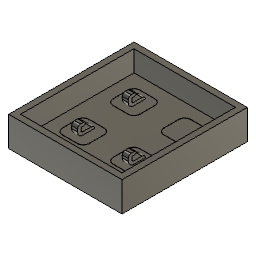
Modular key holder (Autodesk Fusion 360 design; units mm, degrees)
Autodesk Fusion 360 part; units mm, degrees
sketch "Sketch1" plane through (0, 0, 0) normal (0, 0, 1) x (1, 0, 0)
  line L0 (0, 0) -> (190, 0)
  line L1 (190, 0) -> (190, 210)
  line L2 (190, 210) -> (0, 210)
  line L3 (0, 210) -> (0, 0)
  line L4 (10, 10) -> (180, 10)
  line L5 (180, 10) -> (180, 200)
  line L6 (180, 200) -> (10, 200)
  line L7 (10, 200) -> (10, 10)
  dimension "d1" = 190
  dimension "d2" = 210
  dimension "d3" = -10
  constraint horizontal L0
  constraint vertical L1
  constraint horizontal L2
  constraint vertical L3
  constraint coincident L0.start L3.end
  measures "d1" distance of L0.start L0.end
  measures "d2" distance of L0.start L2.end
extrude "Extrude1" add sketch "Sketch1" along normal blind 50 makes body 1
extrude "Extrude2" add sketch "Sketch1" along normal blind 15 contours L4 L5 L6 L7 bodies 1
sketch "Sketch2" plane through (0, 0, 0) normal (0, 0, -1) x (1, 0, 0)
  line L0 (0, 0) -> (0, -210)
  line L1 (0, -210) -> (190, -210)
  line L2 (190, -210) -> (190, 0)
  line L3 (190, 0) -> (0, 0)
  line L4 (170, -160) -> (20, -160)
  line L5 (20, -160) -> (20, -145)
  line L6 (20, -145) -> (170, -145)
  line L7 (170, -145) -> (170, -160)
  dimension "d10" = 150
  dimension "d11" = 15
  constraint horizontal L4
  constraint vertical L5
  constraint horizontal L6
  constraint vertical L7
  measures "d10" distance of L4.start L4.end
  measures "d11" distance of L4.start L6.end
extrude "Extrude3" cut sketch "Sketch2" against normal blind 7 contours L4 L5 L6 L7 bodies 1
sketch "Sketch3" plane through (0, 0, 7) normal (0, 0, -1) x (1, 0, 0)
  line L0 (170, -145) -> (20, -145)
  line L1 (20, -145) -> (20, -160)
  line L2 (20, -160) -> (170, -160)
  line L3 (170, -160) -> (170, -145)
  spline S0 degree 2 poles (16.5, -160) (20.152, -154.0538) (23.5, -160) knots 0 0 0 1.133962 1.133962 1.133962 weights 1 3 1
  spline S1 degree 2 poles (23.0217, -160) (26.6738, -154.0538) (30.0217, -160) knots 0 0 0 1.133962 1.133962 1.133962 weights 1 3 1
  spline S2 degree 2 poles (29.5435, -160) (33.1955, -154.0538) (36.5435, -160) knots 0 0 0 1.133962 1.133962 1.133962 weights 1 3 1
  spline S3 degree 2 poles (36.0652, -160) (39.7173, -154.0538) (43.0652, -160) knots 0 0 0 1.133962 1.133962 1.133962 weights 1 3 1
  spline S4 degree 2 poles (42.587, -160) (46.239, -154.0538) (49.587, -160) knots 0 0 0 1.133962 1.133962 1.133962 weights 1 3 1
  spline S5 degree 2 poles (49.1087, -160) (52.7607, -154.0538) (56.1087, -160) knots 0 0 0 1.133962 1.133962 1.133962 weights 1 3 1
  spline S6 degree 2 poles (55.6304, -160) (59.2825, -154.0538) (62.6304, -160) knots 0 0 0 1.133962 1.133962 1.133962 weights 1 3 1
  spline S7 degree 2 poles (62.1522, -160) (65.8042, -154.0538) (69.1522, -160) knots 0 0 0 1.133962 1.133962 1.133962 weights 1 3 1
  spline S8 degree 2 poles (68.6739, -160) (72.326, -154.0538) (75.6739, -160) knots 0 0 0 1.133962 1.133962 1.133962 weights 1 3 1
  spline S9 degree 2 poles (75.1957, -160) (78.8477, -154.0538) (82.1957, -160) knots 0 0 0 1.133962 1.133962 1.133962 weights 1 3 1
  spline S10 degree 2 poles (81.7174, -160) (85.3694, -154.0538) (88.7174, -160) knots 0 0 0 1.133962 1.133962 1.133962 weights 1 3 1
  spline S11 degree 2 poles (88.2391, -160) (91.8912, -154.0538) (95.2391, -160) knots 0 0 0 1.133962 1.133962 1.133962 weights 1 3 1
  spline S12 degree 2 poles (94.7609, -160) (98.4129, -154.0538) (101.7609, -160) knots 0 0 0 1.133962 1.133962 1.133962 weights 1 3 1
  spline S13 degree 2 poles (101.2826, -160) (104.9347, -154.0538) (108.2826, -160) knots 0 0 0 1.133962 1.133962 1.133962 weights 1 3 1
  spline S14 degree 2 poles (107.8043, -160) (111.4564, -154.0538) (114.8043, -160) knots 0 0 0 1.133962 1.133962 1.133962 weights 1 3 1
  spline S15 degree 2 poles (114.3261, -160) (117.9781, -154.0538) (121.3261, -160) knots 0 0 0 1.133962 1.133962 1.133962 weights 1 3 1
  spline S16 degree 2 poles (120.8478, -160) (124.4999, -154.0538) (127.8478, -160) knots 0 0 0 1.133962 1.133962 1.133962 weights 1 3 1
  spline S17 degree 2 poles (127.3696, -160) (131.0216, -154.0538) (134.3696, -160) knots 0 0 0 1.133962 1.133962 1.133962 weights 1 3 1
  spline S18 degree 2 poles (133.8913, -160) (137.5433, -154.0538) (140.8913, -160) knots 0 0 0 1.133962 1.133962 1.133962 weights 1 3 1
  spline S19 degree 2 poles (140.413, -160) (144.0651, -154.0538) (147.413, -160) knots 0 0 0 1.133962 1.133962 1.133962 weights 1 3 1
  spline S20 degree 2 poles (146.9348, -160) (150.5868, -154.0538) (153.9348, -160) knots 0 0 0 1.133962 1.133962 1.133962 weights 1 3 1
  spline S21 degree 2 poles (153.4565, -160) (157.1086, -154.0538) (160.4565, -160) knots 0 0 0 1.133962 1.133962 1.133962 weights 1 3 1
  spline S22 degree 2 poles (159.9783, -160) (163.6303, -154.0538) (166.9783, -160) knots 0 0 0 1.133962 1.133962 1.133962 weights 1 3 1
  spline S23 degree 2 poles (166.5, -160) (170.152, -154.0538) (173.5, -160) knots 0 0 0 1.133962 1.133962 1.133962 weights 1 3 1
  dimension "d18" = 0
  dimension "d19" = -150
extrude "Extrude4" add sketch "Sketch3" along normal blind 2 from surface at 5 contours L2 L3 S22 S23 | L1 L2 S0 S1 | L2 S21 S22 S23 | L2 S22 S23 | L2 S0 S1 S2 | L2 S0 S1 | L2 S20 S21 S22 | L2 S21 S22 | L2 S1 S2 S3 | L2 S1 S2 | L2 S19 S20 S21 | L2 S20 S21 | L2 S2 S3 S4 | L2 S2 S3 | L2 S18 S19 S20 | L2 S19 S20 | L2 S3 S4 S5 | L2 S3 S4 | L2 S17 S18 S19 | L2 S18 S19 | L2 S4 S5 S6 | L2 S4 S5 | L2 S16 S17 S18 | L2 S17 S18 | L2 S5 S6 S7 | L2 S5 S6 | L2 S15 S16 S17 | L2 S16 S17 | L2 S6 S7 S8 | L2 S6 S7 | L2 S14 S15 S16 | L2 S15 S16 | L2 S7 S8 S9 | L2 S7 S8 | L2 S13 S14 S15 | L2 S14 S15 | L2 S8 S9 S10 | L2 S8 S9 | L2 S12 S13 S14 | L2 S13 S14 | L2 S9 S10 S11 | L2 S9 S10 | L2 S11 S12 S13 | L2 S12 S13 | L2 S10 S11 S12 | L2 S10 S11 | L2 S11 S12 bodies 1
sketch "Sketch4" plane through (0, 0, 15) normal (0, 0, 1) x (-1, 0, 0)
  line L0 (-10, -200) -> (-10, -10)
  line L1 (-10, -10) -> (-180, -10)
  line L2 (-180, -10) -> (-180, -200)
  line L3 (-180, -200) -> (-10, -200)
  line L4 (-40, -180) -> (-65, -180)
  line L5 (-75, -170) -> (-75, -145)
  line L6 (-65, -135) -> (-40, -135)
  line L7 (-30, -145) -> (-30, -170)
  line L8 (-150, -180) -> (-125, -180)
  line L9 (-115, -170) -> (-115, -145)
  line L10 (-125, -135) -> (-150, -135)
  line L11 (-160, -145) -> (-160, -170)
  line L12 (-40, -95) -> (-65, -95)
  line L13 (-75, -85) -> (-75, -60)
  line L14 (-65, -50) -> (-40, -50)
  line L15 (-30, -60) -> (-30, -85)
  line L16 (-150, -95) -> (-125, -95)
  line L17 (-115, -85) -> (-115, -60)
  line L18 (-160, -60) -> (-160, -85)
  line L19 (-125, -50) -> (-150, -50)
  arc A0 (-40, -180) -> (-30, -170) centre (-40, -170) ccw
  arc A1 (-75, -170) -> (-65, -180) centre (-65, -170) ccw
  arc A2 (-65, -135) -> (-75, -145) centre (-65, -145) ccw
  arc A3 (-30, -145) -> (-40, -135) centre (-40, -145) ccw
  arc A4 (-125, -180) -> (-115, -170) centre (-125, -170) ccw
  arc A5 (-160, -170) -> (-150, -180) centre (-150, -170) ccw
  arc A6 (-150, -135) -> (-160, -145) centre (-150, -145) ccw
  arc A7 (-115, -145) -> (-125, -135) centre (-125, -145) ccw
  arc A8 (-125, -95) -> (-115, -85) centre (-125, -85) ccw
  arc A9 (-160, -85) -> (-150, -95) centre (-150, -85) ccw
  arc A10 (-150, -50) -> (-160, -60) centre (-150, -60) ccw
  arc A11 (-115, -60) -> (-125, -50) centre (-125, -60) ccw
  arc A12 (-65, -50) -> (-75, -60) centre (-65, -60) ccw
  arc A13 (-30, -60) -> (-40, -50) centre (-40, -60) ccw
  arc A14 (-75, -85) -> (-65, -95) centre (-65, -85) ccw
  arc A15 (-40, -95) -> (-30, -85) centre (-40, -85) ccw
  point P0 (-30, -180)
  point P1 (-75, -180)
  point P2 (-30, -135)
  point P3 (-160, -180)
  point P4 (-115, -180)
  point P5 (-160, -135)
  point P6 (-160, -95)
  point P7 (-30, -50)
  point P8 (-115, -95)
  point P9 (-160, -50)
  point P10 (-30, -95)
  point P11 (-75, -95)
  dimension "d27" = 45
  dimension "d28" = 45
  dimension "d29" = 45
  dimension "d30" = 45
  dimension "d31" = 45
  dimension "d32" = 45
  dimension "d33" = 45
  dimension "d34" = 45
  dimension "d35" = 10
  constraint horizontal L4
  constraint vertical L5
  constraint horizontal L6
  constraint vertical L7
  constraint horizontal L8
  constraint vertical L9
  constraint horizontal L10
  constraint vertical L11
  constraint horizontal L12
  constraint vertical L13
  constraint horizontal L14
  constraint vertical L15
  constraint horizontal L16
  constraint vertical L17
  constraint horizontal L19
  constraint vertical L18
  constraint coincident P0 L4
  constraint coincident P0 L7
  constraint tangent L4 A0
  constraint tangent L7 A0
  constraint coincident P1 L4
  constraint coincident P1 L5
  constraint tangent L4 A1
  constraint tangent L5 A1
  constraint equal A0 A1
  constraint tangent L5 A2
  constraint tangent L6 A2
  constraint equal A0 A2
  constraint coincident P2 L6
  constraint coincident P2 L7
  constraint tangent L6 A3
  constraint tangent L7 A3
  constraint equal A0 A3
  constraint coincident P4 L8
  constraint coincident P4 L9
  constraint tangent L8 A4
  constraint tangent L9 A4
  constraint equal A0 A4
  constraint coincident P3 L8
  constraint coincident P3 L11
  constraint tangent L8 A5
  constraint tangent L11 A5
  constraint equal A0 A5
  constraint coincident P5 L10
  constraint coincident P5 L11
  constraint tangent L10 A6
  constraint tangent L11 A6
  constraint equal A0 A6
  constraint tangent L9 A7
  constraint tangent L10 A7
  constraint equal A0 A7
  constraint coincident P8 L16
  constraint coincident P8 L17
  constraint tangent L16 A8
  constraint tangent L17 A8
  constraint equal A0 A8
  constraint coincident P6 L16
  constraint coincident P6 L18
  constraint tangent L16 A9
  constraint tangent L18 A9
  constraint equal A0 A9
  constraint coincident P9 L18
  constraint coincident P9 L19
  constraint tangent L18 A10
  constraint tangent L19 A10
  constraint equal A0 A10
  constraint tangent L17 A11
  constraint tangent L19 A11
  constraint equal A0 A11
  constraint tangent L13 A12
  constraint tangent L14 A12
  constraint equal A0 A12
  constraint coincident P7 L14
  constraint coincident P7 L15
  constraint tangent L14 A13
  constraint tangent L15 A13
  constraint equal A0 A13
  constraint coincident P11 L12
  constraint coincident P11 L13
  constraint tangent L12 A14
  constraint tangent L13 A14
  constraint equal A0 A14
  constraint coincident P10 L12
  constraint coincident P10 L15
  constraint tangent L12 A15
  constraint tangent L15 A15
  constraint equal A0 A15
  measures "d27" distance of P0 P1
  measures "d28" distance of P0 P2
  measures "d29" distance of P3 P4
  measures "d30" distance of P3 P5
  measures "d31" distance of P10 P11
  measures "d32" distance of P7 P10
  measures "d33" distance of P6 P8
  measures "d34" distance of P6 P9
  measures "d35" radius of A0
extrude "Extrude5" cut sketch "Sketch4" against normal blind 7 contours L4 L5 L6 L7 A0 A1 A2 A3 | L8 L9 L10 L11 A4 A5 A6 A7 | L12 L13 L14 L15 A12 A13 A14 A15 | L16 L17 L18 L19 A8 A9 A10 A11 bodies 1
sketch "Sketch5" plane through (0, 0, 7) normal (0, 0, -1) x (1, 0, 0)
  line L0 (170, -145) -> (20, -145)
  line L1 (20, -145) -> (20, -160)
  line L2 (20, -160) -> (170, -160)
  line L3 (170, -160) -> (170, -145)
sketch "Sketch7" plane through (0, 0, 8) normal (0, 0, 1) x (-1, 0, 0)
  arc A0 (-40, -180) -> (-30, -170) centre (-40, -170) ccw
  line L0 (-30, -170) -> (-30, -145)
  arc A1 (-30, -145) -> (-40, -135) centre (-40, -145) ccw
  line L1 (-40, -135) -> (-65, -135)
  arc A2 (-65, -135) -> (-75, -145) centre (-65, -145) ccw
  line L2 (-75, -145) -> (-75, -170)
  arc A3 (-75, -170) -> (-65, -180) centre (-65, -170) ccw
  line L3 (-65, -180) -> (-40, -180)
  circle A4 centre (-37, -57) radius 2.5
  circle A5 centre (-68, -57) radius 2.5
  circle A6 centre (-68, -87) radius 2.5
  circle A7 centre (-37, -87) radius 2.5
  circle A8 centre (-37, -172) radius 2.5
  circle A9 centre (-37, -142) radius 2.5
  circle A10 centre (-68, -142) radius 2.5
  circle A11 centre (-68, -172) radius 2.5
  circle A12 centre (-122, -172) radius 2.5
  circle A13 centre (-153, -172) radius 2.5
  circle A14 centre (-153, -142) radius 2.5
  circle A15 centre (-122, -142) radius 2.5
  circle A16 centre (-122, -87) radius 2.5
  circle A17 centre (-122, -57) radius 2.5
  circle A18 centre (-153, -57) radius 2.5
  circle A19 centre (-153, -87) radius 2.5
  dimension "d38" = 5
  dimension "d39" = 5
  dimension "d40" = 5
  dimension "d41" = 5
  dimension "d42" = 5
  dimension "d43" = 5
  dimension "d44" = 5
  dimension "d45" = 5
  dimension "d46" = 5
  dimension "d47" = 5
  dimension "d48" = 5
  dimension "d49" = 5
  dimension "d50" = 5
  dimension "d51" = 5
  dimension "d52" = 5
  dimension "d53" = 5
  measures "d38" diameter of A4
  measures "d39" diameter of A5
  measures "d40" diameter of A7
  measures "d41" diameter of A6
  measures "d42" diameter of A9
  measures "d43" diameter of A10
  measures "d44" diameter of A8
  measures "d45" diameter of A11
  measures "d46" diameter of A17
  measures "d47" diameter of A18
  measures "d48" diameter of A16
  measures "d49" diameter of A19
  measures "d50" diameter of A15
  measures "d51" diameter of A14
  measures "d52" diameter of A12
  measures "d53" diameter of A13
extrude "Extrude6" cut sketch "Sketch7" against normal blind 2 from surface at -0.5 contours A4 | A5 | A6 | A7 | A8 | A9 | A10 | A11 | A12 | A13 | A14 | A15 | A16 | A17 | A18 | A19 bodies 1
sketch "Sketch8" plane through (0, 0, 8) normal (0, 0, 1) x (-1, 0, 0)
  arc A0 (-40, -180) -> (-30, -170) centre (-40, -170) ccw
  line L0 (-30, -170) -> (-30, -145)
  arc A1 (-30, -145) -> (-40, -135) centre (-40, -145) ccw
  line L1 (-40, -135) -> (-65, -135)
  arc A2 (-65, -135) -> (-75, -145) centre (-65, -145) ccw
  line L2 (-75, -145) -> (-75, -170)
  arc A3 (-75, -170) -> (-65, -180) centre (-65, -170) ccw
  line L3 (-65, -180) -> (-40, -180)
  line L4 (-30.25, -170) -> (-30.25, -145)
  arc A4 (-30.25, -145) -> (-40, -135.25) centre (-40, -145) ccw
  line L5 (-40, -135.25) -> (-65, -135.25)
  arc A5 (-65, -135.25) -> (-74.75, -145) centre (-65, -145) ccw
  line L6 (-74.75, -145) -> (-74.75, -170)
  arc A6 (-74.75, -170) -> (-65, -179.75) centre (-65, -170) ccw
  line L7 (-65, -179.75) -> (-40, -179.75)
  arc A7 (-40, -179.75) -> (-30.25, -170) centre (-40, -170) ccw
  circle A8 centre (-37, -142) radius 2.5
  circle A9 centre (-68, -142) radius 2.5
  circle A10 centre (-68, -172) radius 2.5
  circle A11 centre (-37, -172) radius 2.5
  dimension "d57" = -0.25
  dimension "d58" = 5
  dimension "d59" = 5
  dimension "d60" = 5
  dimension "d61" = 5
  measures "d58" diameter of A8
  measures "d59" diameter of A9
  measures "d60" diameter of A10
  measures "d61" diameter of A11
extrude "Extrude7" add sketch "Sketch8" sketch "Sketch7" along normal blind 6.75 from surface at 0.25 separate body contours L4 A4 L5 A5 L6 A6 L7 A7 | A8 of sketch 2 contours A8 | A10 | A11 makes body 2
extrude "Extrude8" cut sketch "Sketch7" along normal blind 2 from surface at 0.5 contours A8 | A9 | A10 | A11 bodies 2
sketch "Sketch9" plane through (0, 0, 15) normal (0, 0, 1) x (-1, 0, 0)
  arc A0 (-40, -179.75) -> (-30.25, -170) centre (-40, -170) ccw
  line L0 (-30.25, -170) -> (-30.25, -145)
  arc A1 (-30.25, -145) -> (-40, -135.25) centre (-40, -145) ccw
  line L1 (-40, -135.25) -> (-65, -135.25)
  arc A2 (-65, -135.25) -> (-74.75, -145) centre (-65, -145) ccw
  line L2 (-74.75, -145) -> (-74.75, -170)
  arc A3 (-74.75, -170) -> (-65, -179.75) centre (-65, -170) ccw
  line L3 (-65, -179.75) -> (-40, -179.75)
  line L4 (-47.55, -172.8615) -> (-57.55, -172.8615)
  line L5 (-57.55, -172.8615) -> (-57.55, -140.9006)
  line L6 (-57.55, -140.9006) -> (-47.55, -140.9006)
  line L7 (-47.55, -140.9006) -> (-47.55, -172.8615)
  constraint horizontal L4
  constraint vertical L5
  constraint horizontal L6
  constraint vertical L7
extrude "Extrude9" add sketch "Sketch9" along normal blind 18 contours L4 L5 L6 L7 bodies 2
sketch "Sketch10" plane through (57.55, 0, 0) normal (1, 0, 0) x (0, 1, 0)
  line L0 (140.9006, 15) -> (172.8615, 15)
  line L1 (172.8615, 15) -> (172.8615, 33)
  line L2 (172.8615, 33) -> (140.9006, 33)
  line L3 (140.9006, 33) -> (140.9006, 15)
  line L4 (166, 20) -> (151.25, 20)
  line L5 (152, 15) -> (171.9161, 15)
  line L6 (149, 22.25) -> (149, 27)
  line L7 (148, 33) -> (153.14, 33)
  line L8 (153.2103, 28) -> (150, 28)
  line L9 (143, 28) -> (143, 24)
  arc A0 (148, 33) -> (143, 28) centre (148, 28) ccw
  arc A1 (153.2103, 28) -> (155.7841, 28.938) centre (153.2103, 32) ccw
  arc A2 (155.8544, 31.938) -> (153.14, 33) centre (153.14, 29) ccw
  arc A3 (155.7841, 28.938) -> (155.8544, 31.938) centre (154.4972, 30.469) ccw
  arc A4 (150, 28) -> (149, 27) centre (150, 27) ccw
  arc A5 (149, 22.25) -> (151.25, 20) centre (151.25, 22.25) ccw
  arc A6 (143, 24) -> (152, 15) centre (152, 24) ccw
  arc A7 (171.9161, 15) -> (166, 20) centre (166, 14) ccw
  dimension "d71" = 4
  dimension "d72" = 2
  dimension "d73" = 1
  dimension "d74" = 2.25
  dimension "d75" = 9
  dimension "d76" = 6
  constraint horizontal L4
  constraint horizontal L5
  constraint vertical L6
  constraint perpendicular L6 L8
  constraint perpendicular L5 L9
  constraint tangent L7 A0
  constraint tangent L9 A0
  constraint tangent L8 A1
  constraint tangent L7 A2
  constraint equal A1 A2
  constraint tangent A1 A3
  constraint tangent A2 A3
  constraint tangent L6 A4
  constraint tangent L8 A4
  constraint tangent L6 A5
  constraint tangent L4 A5
  constraint tangent L5 A6
  constraint tangent L9 A6
  constraint tangent L4 A7
  constraint coincident L0 L5.end
  measures "d71" radius of A1
  measures "d72" radius of A3
  measures "d73" radius of A4
  measures "d74" radius of A5
  measures "d75" radius of A6
  measures "d76" radius of A7
extrude "Extrude10" cut sketch "Sketch10" against normal blind 10 contours L0 L2 L3 L9 A0 A6 | L0 L1 L2 L4 L6 L8 A1 A2 A3 A4 A5 A7 bodies 2
copy_body "CopyPasteBodies1" bodies 2 makes body 3
move_body "Move1" bodies 3 to x (1, 0, 0) y (0, 1, 0) z (0, 0, 1) at (85, 0, 0)
copy_body "CopyPasteBodies2" bodies 3 makes body 4
move_body "Move2" bodies 4 to x (1, 0, 0) y (0, 1, 0) z (0, 0, 1) at (0, -85, 0)
copy_body "CopyPasteBodies3" bodies 3 makes body 5
move_body "Move3" bodies 5 to x (1, 0, 0) y (0, 1, 0) z (0, 0, 1) at (-85, -85, 0)
extrude "Extrude11" cut 1 faces at (142.55, 163.3054, 16.6667) along direction (-1, 0, 0) blind 10 on bodies 3 bodies 3
named bodies: "Wall Base", "Hook module", "Blank module", "Hook module (1)", "Hook module (2)"
